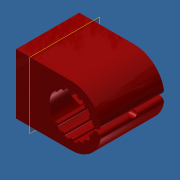
# Autodesk Inventor part: claww
Saved by Autodesk Inventor 2015 (Build 190159000, 159)
## iProperties
Created: 2018-12-07
Part Number: claww
Material: Generic
Document SubType Name: Modeling
Designer: gabriel
Density: 1 g/cm^3
Appearance: Default
Author: gabriel
Autodesk Inventor part; units mm, degrees
ref_plane "YZ Plane" through (0, 0, 0) normal (1, 0, 0) x (0, 1, 0)
ref_plane "XZ Plane" through (0, 0, 0) normal (0, 1, 0) x (-1, 0, 0)
ref_plane "XY Plane" through (0, 0, 0) normal (0, 0, 1) x (1, 0, 0)
sketch "Sketch1" plane through (0, 0, 0) normal (0, 0, 1) x (1, 0, 0)
  arc A0 (4.0641, 0.1774) -> (4.0641, -0.1774) centre (0, 0) ccw
  arc A1 (5.6501, 0.2467) -> (5.6501, -0.2467) centre (0, 0) ccw
  line L0 (4.0641, -0.1774) -> (5.6501, -0.2467)
  line L1 (4.0641, 0.1774) -> (5.6501, 0.2467)
  dimension "d0" = 8.1359
  dimension "d13" = 5
  dimension "d26" = 1.5875
  constraints: 4 end point, 4 point on circle, 2 centre point, 2 coincident, 2 point on line, 1 vertical alignment
  measures "d0" diameter of A0
  measures "d13" angle of L0 L1
  measures "d26" radial gap between concentric circles of A0 A1
extrude "Extrusion3" add sketch "Sketch1" along normal blind 11.9062
fillet "Fillet4" radius 0.7937 4 edges at (5.6501, 0.2467, 5.9531) (4.0641, 0.1774, 5.9531) (4.0641, -0.1774, 5.9531) (5.6501, -0.2467, 5.9531)
sketch "Sketch4" plane through (0, 0, 11.9062) normal (0, 0, 1) x (1, 0, 0)
  arc A0 (5.534, 1.1658) -> (5.534, -1.1658) centre (0, 0) ccw projected
  arc A1 (0, 5.6555) -> (0, -5.6555) centre (0, 0) ccw
  line L0 (0, 5.6555) -> (-10.3791, 5.6555)
  line L1 (-10.3791, 5.6555) -> (-10.3791, -5.6555)
  line L2 (0, -5.6555) -> (-10.3791, -5.6555)
  dimension "d192" = 10.3791
  constraints: 6 end point, 4 point on circle, 1 centre point, 1 concentric, 1 horizontal, 1 parallel, 1 perpendicular, 1 tangent, 1 vertical alignment
  measures "d192" distance of L2.start L1.end
extrude "Extrusion5" add sketch "Sketch4" against normal up to surface (11.9062 mm away)
sketch "Sketch8" plane through (0, 0, 11.9062) normal (0, 0, 1) x (1, 0, 0)
  arc A0 (3.9806, 0.8386) -> (3.9806, -0.8386) centre (0, 0) ccw projected
  circle A1 centre (0, 4.068) radius 0.3969
  circle A2 centre (0, -4.068) radius 0.3969
  circle A3 centre (-1.5567, 3.7583) radius 0.3969
  circle A4 centre (-1.5567, -3.7583) radius 0.3969
  circle A5 centre (-2.8765, 2.8765) radius 0.3969
  circle A6 centre (-2.8765, -2.8765) radius 0.3969
  circle A7 centre (1.5567, 3.7583) radius 0.3969
  circle A8 centre (1.5567, -3.7583) radius 0.3969
  circle A9 centre (2.8765, 2.8765) radius 0.3969
  circle A10 centre (2.8765, -2.8765) radius 0.3969
  arc A11 (3.9806, 0.8386) -> (3.9806, -0.8386) centre (0, 0) ccw projected
  circle A12 centre (3.7583, 1.5567) radius 0.3969
  circle A13 centre (3.7583, -1.5567) radius 0.3969
  point P0 (4.7625, 0)
  dimension "d71" = 4.7625
  dimension "d72" = 0.7937
  dimension "d74" = 0.7937
  dimension "d75" = 0.7937
  dimension "d76" = 22.5
  dimension "d77" = 0.7937
  dimension "d78" = 22.5
  dimension "d110" = 0.7937
  dimension "d111" = 0.7937
  dimension "d112" = 22.5
  dimension "d113" = 22.5
  dimension "d158" = 0.7937
  dimension "d159" = 0.7937
  dimension "d160" = 22.5
  dimension "d161" = 22.5
  dimension "d165" = 0.7937
  dimension "d166" = 0.7937
  dimension "d167" = 22.5
  dimension "d168" = 22.5
  dimension "d171" = 22.5
  dimension "d172" = 0.7937
  dimension "d173" = 0.7937
  dimension "d174" = 22.5
  dimension "d191" = 45
  constraints: 12 centre point, 2 point on circle, 1 horizontal alignment, 1 vertical alignment, 13 other
  measures "d71" distance of point (0, 0) point (4.763, 0)
  measures "d72" diameter of A1
  measures "d74" diameter of A2
  measures "d75" diameter of A3
  measures "d77" diameter of A4
  measures "d110" diameter of A5
  measures "d111" diameter of A6
  measures "d158" diameter of A7
  measures "d159" diameter of A8
  measures "d165" diameter of A9
  measures "d166" diameter of A10
  measures "d172" diameter of A12
  measures "d173" diameter of A13
sketch "Sketch22" plane through (-10.3791, -5.6555, 11.9062) normal (-1, 0, 0) x (0, 0, 1)
  line L0 (-4.9752, 8.0367) -> (-3.6004, 5.6555)
  line L1 (-3.6004, 5.6555) -> (-4.9752, 3.2742)
  line L2 (-4.9752, 3.2742) -> (-7.7248, 3.2742)
  line L3 (-7.7248, 3.2742) -> (-9.0996, 5.6555)
  line L4 (-9.0996, 5.6555) -> (-7.7248, 8.0367)
  line L5 (-7.7248, 8.0367) -> (-4.9752, 8.0367)
  line L6 (0, 11.3109) -> (-11.9062, 11.3109) projected
  line L7 (0, 11.3109) -> (0, 0) projected
  point P0 (-11.9062, 5.6555)
  point P1 (-6.35, 5.6555)
  dimension "d145" = 4.7625
  dimension "d146" = 5.6555
  dimension "d147" = 6.35
  constraints: 12 end point, 1 horizontal, 13 other
  measures "d145" distance between parallel lines of L2 L5
  measures "d146" distance from line of L6 point (-6.35, 5.655)
  measures "d147" distance from line of L7 point (-6.35, 5.655)
extrude "Extrusion28" cut sketch "Sketch22" against normal up to surface
extrude "Extrusion36" add sketch "Sketch8" against normal up to surface (11.9062 mm away)
ref_plane "Work Plane3" through (-7.2041, -5.6555, 11.9062) normal (-1, 0, 0) x (0, 0, 1)
sketch "Sketch28" plane through (-7.2041, -5.6555, 11.9062) normal (-1, 0, 0) x (0, 0, 1)
  line L0 (-4.9752, 8.0367) -> (-3.6004, 5.6555)
  line L1 (-3.6004, 5.6555) -> (-4.9752, 3.2742)
  line L2 (-4.9752, 3.2742) -> (-7.7248, 3.2742)
  line L3 (-7.7248, 3.2742) -> (-9.0996, 5.6555)
  line L4 (-9.0996, 5.6555) -> (-7.7248, 8.0367)
  line L5 (-7.7248, 8.0367) -> (-4.9752, 8.0367)
  line L6 (-7.7248, 8.0367) -> (-4.9752, 8.0367) projected
  line L7 (-9.0996, 5.6555) -> (-7.7248, 8.0367) projected
  line L8 (-3.6004, 5.6555) -> (-4.9752, 3.2742) projected
  circle A0 centre (-6.35, 5.6555) radius 1.5875
  point P0 (-11.9062, 5.6555)
  dimension "d194" = 3.175
  constraints: 12 end point, 3 collinear, 1 centre point, 1 coincident, 13 other
  measures "d194" diameter of A0
extrude "Extrusion37" add sketch "Sketch28" against normal blind 1.5875
sketch "Sketch29" plane through (-7.2041, -5.6555, 11.9062) normal (-1, 0, 0) x (0, 0, 1)
  circle A0 centre (-6.35, 5.6555) radius 1.5875 projected
  circle A1 centre (-6.35, 5.6555) radius 0.7937
  point P0 (-11.9062, 5.6555)
  dimension "d197" = 1.5875
  constraints: 1 centre point, 1 coincident
  measures "d197" diameter of A1
extrude "Extrusion38" cut sketch "Sketch29" against normal through all contours A1
equation "\"d72\" = d75"
equation "\"d74\" = d75"
equation "\"d77\" = d75"
equation "\"d110\" = d75"
equation "\"d111\" = d75"
equation "\"d158\" = d75"
equation "\"d159\" = d75"
equation "\"d165\" = d75"
equation "\"d166\" = d75"
body "Solid2"
